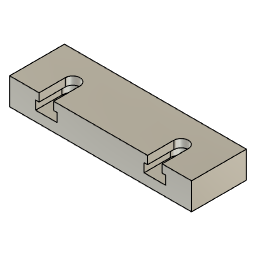
Quick-Change Soft Jaws (Autodesk Fusion 360 design; units mm, degrees)
Autodesk Fusion 360 part; units mm, degrees
sketch "Sketch1" plane through (0, 0, 0) normal (0, 0, 1) x (1, 0, 0)
  line L0 (82.55, 24.892) -> (-82.55, 24.892)
  line L1 (-82.55, 24.892) -> (-82.55, -24.892)
  line L2 (-82.55, -24.892) -> (82.55, -24.892)
  line L3 (82.55, -24.892) -> (82.55, 24.892)
  line L4 (82.55, 24.892) -> (-82.55, -24.892) construction
  line L5 (-82.55, 24.892) -> (82.55, -24.892) construction
  circle A0 centre (-49.2125, -1.016) radius 3.9688
  circle A1 centre (49.2125, -1.016) radius 3.9688
  line L6 (-39.4335, -1.016) -> (-39.4335, -24.892)
  line L7 (-58.9915, -1.016) -> (-58.9915, -24.892)
  line L8 (39.4335, -1.016) -> (39.4335, -24.892)
  line L9 (58.9915, -1.016) -> (58.9915, -24.892)
  arc A2 (-39.4335, -1.016) -> (-58.9915, -1.016) centre (-49.2125, -1.016) ccw
  arc A3 (58.9915, -1.016) -> (39.4335, -1.016) centre (49.2125, -1.016) ccw
  line L10 (0, 24.892) -> (0, -24.892) construction
  circle A4 centre (-49.2125, -1.016) radius 6.604
  circle A5 centre (49.2125, -1.016) radius 6.604
  line L11 (-42.6085, -1.016) -> (-42.6085, -24.892)
  line L12 (-55.8165, -1.016) -> (-55.8165, -24.892)
  line L13 (42.6085, -1.016) -> (42.6085, -24.892)
  line L14 (55.8165, -1.016) -> (55.8165, -24.892)
  point P0 (-49.2125, -1.016)
  point P1 (49.2125, -1.016)
  dimension "d1" = 165.1
  dimension "d2" = 49.784
  dimension "d3" = 7.9375
  dimension "d4" = 7.9375
  dimension "d5" = 98.425
  dimension "d9" = 23.876
  dimension "d10" = 19.558
  dimension "d11" = 19.558
  dimension "d16" = 23.876
  dimension "d17" = 49.2125
  dimension "d19" = 13.208
  dimension "d20" = 13.208
  constraint perpendicular L0 L1
  constraint parallel L0 L2
  constraint parallel L1 L3
  constraint horizontal L0
  constraint coincident L4 origin
  constraint coincident L5 origin
  constraint coincident P0 A0.centre
  constraint coincident P1 A1.centre
  constraint concentric A0 A2
  constraint coincident L2 L6.end
  constraint tangent L6 A2
  constraint perpendicular L2 L6
  constraint coincident L2 L7.end
  constraint tangent L7 A2
  constraint perpendicular L2 L7
  constraint coincident L2 L8.end
  constraint tangent L8 A3
  constraint perpendicular L2 L8
  constraint coincident L2 L9.end
  constraint tangent L9 A3
  constraint perpendicular L2 L9
  constraint midpoint L0 L10.start
  constraint midpoint L2 L10.end
  constraint concentric A1 A5
  constraint coincident A4 L11.start
  constraint coincident L2 L11.end
  constraint perpendicular L2 L11
  constraint tangent A4 L11
  constraint coincident A4 L12.start
  constraint coincident L2 L12.end
  constraint perpendicular L2 L12
  constraint tangent A4 L12
  constraint coincident A5 L13.start
  constraint coincident L2 L13.end
  constraint perpendicular L2 L13
  constraint coincident A5 L14.start
  constraint coincident L2 L14.end
  constraint perpendicular L2 L14
  constraint tangent A5 L14
  constraint tangent A5 L13
  measures "d1" distance of L1.end L2.end
  measures "d2" distance of L0.end L1.end
  measures "d3" diameter of A0
  measures "d4" diameter of A1
  measures "d5" distance of P0 P1
  measures "d9" distance of L2 P0
  measures "d10" diameter of A2
  measures "d11" diameter of A3
  measures "d16" distance of L2 P1
  measures "d17" distance of P1 L10
  measures "d19" diameter of A4
  measures "d20" diameter of A5
extrude "Extrude1" add sketch "Sketch1" against normal blind 24.384
extrude "Extrude2" cut sketch "Sketch1" against normal blind 15.24 contours L2 L8 L9 A3 A5 L13 L14 | L2 L6 L7 A2 A4 L11 L12 | L2 A5 L13 L14 | L2 A4 L11 L12 | A5 | A4
extrude "Extrude3" add sketch "Sketch1" against normal blind 7.3025 contours L2 L8 L9 A3 A5 L13 L14 | L2 L6 L7 A2 A4 L11 L12
equation "d2 = 2 in - 0.04 in"
equation "d4 = d3"
equation "d11 = d10"
equation "d12 = -1 in + 0.04 in"
equation "d17 = ( 3.875 / 2 ) * 1 in"
equation "d20 = d19"
named bodies: "QuickChangeSoftJaw"
